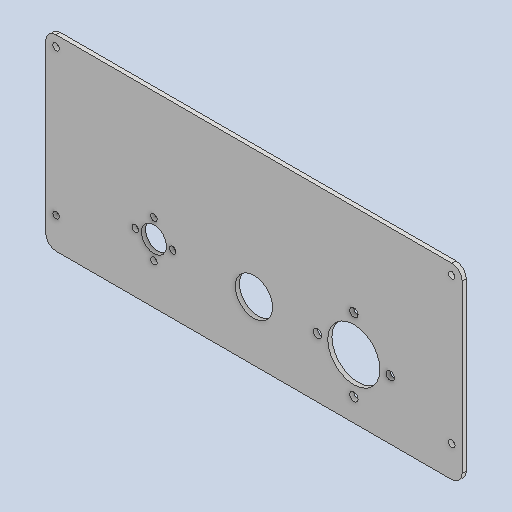
# Autodesk Inventor part: small_plate_shita_motor
Saved by Autodesk Inventor 2025.1 (Build 291241000, 241)
## iProperties
Created: 2024-12-23
Part Number: small_plate_shita_motor
Material: 一般
Document SubType Name: Modeling
Designer: yuki0520
Density: 1 g/cm^3
Appearance: 既定
Author: yuki0520
Autodesk Inventor part; units mm, degrees
ref_plane "YZ Plane" through (0, 0, 0) normal (1, 0, 0) x (0, 1, 0)
ref_plane "XZ Plane" through (0, 0, 0) normal (0, 1, 0) x (-1, 0, 0)
ref_plane "XY Plane" through (0, 0, 0) normal (0, 0, 1) x (1, 0, 0)
derived "small_plate_shita.ipt"
sketch "スケッチ1" plane through (0, 0, 0) normal (0, 0, 1) x (1, 0, 0)
  circle A0 centre (0, -21.5) radius 39
  circle A1 centre (-48, -21.5) radius 6.05
  circle A2 centre (-48, -21.5) radius 9
  line L0 (-95, 35) -> (-95, -35)
  line L1 (-100, -40) -> (-100, 40)
  line L2 (-95, -35) -> (95, -35)
  line L3 (100, -50) -> (-100, -50)
  line L4 (-100, -21.5) -> (100, -21.5)
  line L5 (100, -40) -> (-100, -40)
  line L6 (85, 35) -> (-85, 35)
  line L7 (-100, 0) -> (100, 0)
  line L8 (-85, 40) -> (85, 40)
  line L9 (95, 35) -> (-95, 35)
  line L10 (-100, 40) -> (100, 40)
  line L11 (-100, -40) -> (100, 40) construction
  line L12 (100, -40) -> (-100, 40) construction
  circle A3 centre (48, -4) radius 2.05
  circle A4 centre (30.5, -21.5) radius 2.05
  circle A5 centre (48, -39) radius 2.05
  circle A6 centre (48, -21.5) radius 17.5
  circle A7 centre (65.5, -21.5) radius 2.05
  circle A8 centre (48, -21.5) radius 12.55
  arc A9 (93.4, -35) -> (96.6, -35) centre (95, -35) ccw
  line L13 (85, 40) -> (85, 35)
  line L14 (95, 35) -> (95, 35) construction
  line L15 (0, 0) -> (85, 35)
  line L16 (93.4, 35) -> (93.4, 35)
  line L17 (96.6, 35) -> (96.6, 35)
  arc A10 (93.4, 35) -> (96.6, 35) centre (95, 35) ccw
  arc A11 (96.6, -35) -> (93.4, -35) centre (95, -35) ccw
  line L18 (93.4, -35) -> (93.4, -35)
  line L19 (95, -35) -> (95, -35) construction
  arc A12 (96.6, 35) -> (93.4, 35) centre (95, 35) ccw
  line L20 (95, -35) -> (95, 35)
  line L21 (100, 40) -> (100, -40)
  line L22 (95, 35) -> (95, 35) construction
  line L23 (96.6, -35) -> (96.6, -35)
  line L24 (95, -35) -> (95, -35) construction
  line L25 (100, 0) -> (100, -50)
  circle A13 centre (0, -21.5) radius 9
  circle A14 centre (-39, -21.5) radius 1.6
  circle A15 centre (-48, -30.5) radius 1.6
  circle A16 centre (-48, -12.5) radius 1.6
  circle A17 centre (-57, -21.5) radius 1.6
  line L26 (-85, 35) -> (0, 0)
  line L27 (-93.4, -35) -> (-93.4, -35)
  line L28 (-95, -35) -> (-95, -35) construction
  line L29 (-95, -35) -> (-95, -35) construction
  arc A18 (-96.6, -35) -> (-93.4, -35) centre (-95, -35) ccw
  line L30 (-96.6, -35) -> (-96.6, -35)
  line L31 (-85, 35) -> (-85, 40)
  arc A19 (-93.4, -35) -> (-96.6, -35) centre (-95, -35) ccw
  line L32 (-95, 35) -> (-95, 35) construction
  arc A20 (-96.6, 35) -> (-93.4, 35) centre (-95, 35) ccw
  line L33 (-96.6, 35) -> (-96.6, 35)
  arc A21 (-93.4, 35) -> (-96.6, 35) centre (-95, 35) ccw
  line L34 (-95, 35) -> (-95, 35) construction
  line L35 (-93.4, 35) -> (-93.4, 35)
  line L36 (-100, -50) -> (-100, 0)
  circle A22 centre (48, -21.5) radius 9
  point P0 (0, 40)
  point P1 (95, 35)
  point P2 (95, -35)
  point P3 (-95, 45.5475)
  point P4 (48.45, -35)
  point P5 (47.55, -35)
  point P6 (93.4, -35)
  point P7 (93.4, 35)
  point P8 (96.6, 35)
  point P9 (47.55, 0)
  point P10 (48.45, 0)
  point P11 (-93.4, -35)
  point P12 (-96.6, -35)
  point P13 (38.2031, -13.6563)
  point P14 (38.2031, -29.3437)
extrude "押し出し1" add sketch "スケッチ1" along normal blind 2 contours A8 L4 A4 A6 A0 | A0 A6 A3 A7 L4 A8 | A8 L4 A7 A6 L2 A0 | A0 A6 A4 L4 A8 | A6 A4 L4 A13 A14 A0 L7 | A0 L7 L20 L4 A7 A6 A3 | A6 L2 A0 | A0 L2 A14 L4 A13 A4 A6 | L7 L15 A0 | A0 L15 L9 A10 L20 L7 | L2 A6 A5 L5 A0 | A0 L5 L2 | L2 A6 A5 | L15 L26 A0 | A0 L26 L6 L15 | L7 A0 L26 | L20 A10 A12 L9 L13 L10 L21 L7 | L7 L21 L4 L20 | A7 L4 L20 A11 L2 A6 | L5 A5 L25 L3 A0 | A0 L3 L5 | L2 A19 L0 L4 A17 A2 A15 A14 A0 | A0 L5 L1 L4 L0 A19 A18 L2 | L2 A9 A11 L20 L4 L21 L5 A5 A6 | A0 L7 L0 A20 L9 L26 | L6 L31 L8 L13 | A0 A14 A2 A16 A17 L4 L0 L7 | A0 L3 L36 L5 | L9 A21 A20 L0 L7 L1 L10 L31 | L0 L4 L1 L7 | A2 A15 A17 L4 A1 A14 | A14 L4 A1 A17 A2 A16
fillet "フィレット1" radius 5 4 edges at (100, 40, 1) (-100, 40, 1) (100, -50, 1) (-100, -50, 1)
